Autodesk Fusion 360 part; units mm, degrees
(part 10 of 11)
  line L2802 (-0.2526, -65.3771) -> (-0.2373, -65.4277)
  line L2803 (0.0454, -65.5378) -> (0.0706, -65.5685)
  line L2804 (18.12, -173.2625) -> (18.12, -175.4997)
  line L2805 (-0.08, -80.4997) -> (-0.08, -81.4997)
  line L2806 (20.12, -54.8985) -> (20.1186, -54.7804)
  line L2807 (-0.0174, -65.4367) -> (0.0013, -65.4717)
  line L2808 (-0.0459, -65.7366) -> (1.2372, -67.0197)
  line L2809 (7.0807, -66.0997) -> (3.6807, -62.6997)
  line L2810 (19.8859, -25.7366) -> (19.9198, -25.7004)
  line L2811 (9.7152, -6.0997) -> (7.0807, -6.0997)
  line L2812 (19.7422, -174.4019) -> (18.4614, -173.1211)
  line L2813 (9.7152, -6.0997) -> (7.0807, -6.0997)
  line L2814 (19.9841, -25.6166) -> (20.012, -25.5718)
  line L2815 (18.12, -173.2625) -> (18.12, -175.4997)
  line L2816 (19.8878, -25.3633) -> (19.8993, -25.3253)
  line L2817 (19.8574, -54.5626) -> (19.8387, -54.5276)
  line L2818 (19.8993, -25.3253) -> (19.9083, -25.2866)
  line L2819 (19.9148, -25.2474) -> (19.9187, -25.2079)
  line L2820 (7.0807, -66.0997) -> (3.6807, -62.6997)
  line L2821 (20.0926, -54.6222) -> (20.0773, -54.5717)
  line L2822 (20.0773, -25.4277) -> (20.0926, -25.3771)
  line L2823 (17.92, -173.2625) -> (17.92, -175.2997)
  line L2824 (19.8738, -54.5988) -> (19.8574, -54.5626)
  line L2825 (19.7422, -174.4019) -> (18.4614, -173.1211)
  line L2826 (3.6807, -62.6997) -> (1.72, -62.6997)
  line L2827 (19.7694, -174.4308) -> (19.7422, -174.4019)
  line L2828 (19.7946, -25.5378) -> (19.8177, -25.5055)
  line L2829 (19.8878, -54.636) -> (19.8738, -54.5988)
  line L2830 (6.02, -190.1995) -> (6.02, -192.839)
  line L2831 (0.0706, -65.5685) -> (0.0978, -65.5975)
  line L2832 (12.7593, -66.0997) -> (10.127, -66.0997)
  line L2833 (20.1132, -25.2736) -> (20.1186, -25.2189)
  line L2834 (19.8387, -54.5276) -> (19.8177, -54.4938)
  line L2835 (20.0587, -25.4771) -> (20.0773, -25.4277)
  line L2836 (9.7981, -5.8997) -> (7.1635, -5.8997)
  line L2837 (16.1593, -22.6997) -> (12.7593, -26.0997)
  line L2838 (19.8878, -54.636) -> (19.8738, -54.5988)
  line L2839 (19.7946, -25.5378) -> (19.8177, -25.5055)
  line L2840 (6.02, -190.1995) -> (6.02, -192.839)
  line L2841 (1.92, -64.6997) -> (3.2765, -64.6997)
  line L2842 (19.8993, -54.674) -> (19.8878, -54.636)
  line L2843 (19.7422, -25.5975) -> (19.7694, -25.5685)
  line L2844 (0.0706, -65.5685) -> (0.0978, -65.5975)
  line L2845 (19.9187, -25.2079) -> (19.92, -25.0997)
  line L2846 (19.8177, -54.4938) -> (19.7946, -54.4616)
  arc A174 (18.4614, -173.1211) -> (18.12, -173.2625) centre (18.32, -173.2625) ccw
  line L2847 (1.72, -64.4997) -> (3.3593, -64.4997)
  line L2848 (19.8387, -54.5276) -> (19.8177, -54.4938)
  line L2849 (-0.08, -34.8997) -> (-0.08, -45.0997)
  line L2850 (19.9083, -25.2866) -> (19.9148, -25.2474)
  line L2851 (20.1186, -25.2189) -> (20.12, -25.1009)
  line L2852 (20.012, -54.4275) -> (19.9841, -54.3827)
  line L2853 (1.72, -64.4997) -> (3.3593, -64.4997)
  line L2854 (19.8859, -174.2627) -> (18.6028, -172.9797)
  line L2855 (-0.0593, -65.3253) -> (-0.0478, -65.3633)
  line L2856 (19.7694, -25.5685) -> (19.7946, -25.5378)
  line L2857 (19.7694, -174.4308) -> (19.7422, -174.4019)
  line L2858 (19.9148, -54.7519) -> (19.9083, -54.7127)
  arc A175 (18.6028, -172.9797) -> (17.92, -173.2625) centre (18.32, -173.2625) ccw
  line L2859 (3.7635, -62.4997) -> (1.92, -62.4997)
  line L2860 (3.6807, -62.6997) -> (1.72, -62.6997)
  line L2861 (20.1186, -54.7804) -> (20.1132, -54.7258)
  line L2862 (19.92, -54.8997) -> (19.9187, -54.7914)
  line L2863 (7.1635, -65.8997) -> (3.7635, -62.4997)
  line L2864 (19.8738, -54.5988) -> (19.8574, -54.5626)
  line L2865 (19.8738, -25.4005) -> (19.8878, -25.3633)
  line L2866 (20.0369, -54.4741) -> (20.012, -54.4275)
  line L2867 (20.1132, -54.7258) -> (20.1046, -54.6736)
  line L2868 (12.6765, -65.8997) -> (10.0441, -65.8997)
  line L2869 (19.8387, -25.4717) -> (19.8574, -25.4367)
  line L2870 (20.0773, -54.5717) -> (20.0587, -54.5222)
  line L2871 (13.1828, -1.9997) -> (15.22, -1.9997)
  line L2872 (19.8738, -5.4005) -> (19.8878, -5.3633)
  line L2873 (19.8878, -5.3633) -> (19.8993, -5.3253)
  line L2874 (7.0807, -46.0997) -> (3.6807, -42.6997)
  line L2875 (6.02, -7.1603) -> (6.02, -9.7998)
  line L2876 (19.9083, -25.2866) -> (19.9148, -25.2474)
  line L2877 (20.1132, -5.2736) -> (20.1184, -5.221)
  line L2878 (19.8574, -54.5626) -> (19.8387, -54.5276)
  line L2879 (5.82, -9.8826) -> (5.937, -9.9997)
  line L2880 (10.127, -166.0997) -> (9.92, -166.3066)
  line L2881 (13.82, -167.1603) -> (16.4807, -164.4997)
  line L2882 (12.6765, -14.0997) -> (16.0765, -17.4997)
  line L2883 (19.8177, -25.5055) -> (19.8387, -25.4717)
  line L2884 (6.02, -70.1995) -> (6.02, -72.839)
  line L2885 (10.0441, -165.8997) -> (9.92, -166.0238)
  arc A176 (1.3786, -6.8782) -> (1.72, -6.7368) centre (1.52, -6.7368) ccw
  line L2886 (20.0369, -5.5252) -> (20.0587, -5.4771)
  line L2887 (20.0369, -25.5252) -> (20.0587, -25.4771)
  line L2888 (14.02, -167.2432) -> (16.5635, -164.6997)
  line L2889 (6.02, -9.7998) -> (6.2199, -9.9997)
  line L2890 (19.9148, -54.7519) -> (19.9083, -54.7127)
  line L2891 (19.8993, -25.3253) -> (19.9083, -25.2866)
  line L2892 (19.8878, -5.3633) -> (19.8993, -5.3253)
  line L2893 (19.8993, -54.674) -> (19.8878, -54.636)
  line L2894 (13.82, -72.839) -> (13.82, -70.1995)
  line L2895 (6.2199, -9.9997) -> (6.02, -10.1995)
  line L2896 (5.82, -70.1167) -> (5.82, -72.7562)
  line L2897 (19.9148, -25.2474) -> (19.9187, -25.2079)
  line L2898 (9.92, -166.0238) -> (9.7959, -165.8997)
  line L2899 (13.82, -72.839) -> (13.82, -70.1995)
  line L2900 (9.92, -166.3066) -> (9.713, -166.0997)
  line L2901 (6.2199, -9.9997) -> (6.02, -10.1995)
  line L2902 (9.92, -166.3066) -> (9.713, -166.0997)
  line L2903 (20.012, -25.5718) -> (20.0369, -25.5252)
  line L2904 (19.7946, -54.4616) -> (19.7694, -54.4308)
  line L2905 (6.02, -70.1995) -> (6.02, -72.839)
  line L2906 (20.012, -5.5718) -> (20.0369, -5.5252)
  line L2907 (16.0765, -162.4997) -> (12.6765, -165.8997)
  line L2908 (19.8177, -54.4938) -> (19.7946, -54.4616)
  line L2909 (19.8993, -5.3253) -> (19.9083, -5.2866)
  line L2910 (12.7593, -166.0997) -> (10.127, -166.0997)
  line L2911 (19.8177, -25.5055) -> (19.8387, -25.4717)
  line L2912 (5.82, -7.2432) -> (5.82, -9.8826)
  line L2913 (19.8574, -25.4367) -> (19.8738, -25.4005)
  line L2914 (20.1046, -54.6736) -> (20.0926, -54.6222)
  line L2915 (19.8177, -5.5055) -> (19.8387, -5.4717)
  arc A177 (1.3786, -6.8782) -> (1.72, -6.7368) centre (1.52, -6.7368) ccw
  line L2916 (14.02, -72.7562) -> (14.02, -70.1167)
  line L2917 (20.0587, -54.5222) -> (20.0369, -54.4741)
  line L2918 (19.9533, -54.3397) -> (19.9198, -54.2989)
  line L2919 (12.7593, -166.0997) -> (10.127, -166.0997)
  line L2920 (12.7593, -66.0997) -> (10.127, -66.0997)
  line L2921 (19.9148, -5.2474) -> (19.9187, -5.2079)
  line L2922 (19.9187, -54.7914) -> (19.9148, -54.7519)
  line L2923 (16.1593, -162.6997) -> (12.7593, -166.0997)
  line L2924 (5.937, -9.9997) -> (5.82, -10.1167)
  line L2925 (14.3222, -0.1775) -> (13.0414, -1.4582)
  line L2926 (19.8574, -25.4367) -> (19.8738, -25.4005)
  line L2927 (19.9533, -25.6596) -> (19.9841, -25.6166)
  line L2928 (19.9083, -54.7127) -> (19.8993, -54.674)
  arc A178 (1.2372, -7.0197) -> (1.92, -6.7368) centre (1.52, -6.7368) ccw
  line L2929 (19.9198, -25.7004) -> (19.9533, -25.6596)
  line L2930 (19.7946, -5.5378) -> (19.8177, -5.5055)
  line L2931 (19.8387, -25.4717) -> (19.8574, -25.4367)
  line L2932 (19.7422, -54.4019) -> (18.4614, -53.1211)
  line L2933 (19.7694, -5.5685) -> (19.7946, -5.5378)
  line L2934 (19.8859, -5.7366) -> (19.9198, -5.7004)
  line L2935 (20.0587, -5.4771) -> (20.0773, -5.4277)
  line L2936 (20.0926, -25.3771) -> (20.1046, -25.3257)
  line L2937 (20.12, -45.1009) -> (20.12, -34.8985)
  line L2938 (20.0773, -5.4277) -> (20.0926, -5.3771)
  line L2939 (16.1593, -162.6997) -> (12.7593, -166.0997)
  line L2940 (19.8738, -25.4005) -> (19.8878, -25.3633)
  line L2941 (13.82, -172.839) -> (13.82, -170.1995)
  line L2942 (0.0013, -5.4717) -> (0.0223, -5.5055)
  line L2943 (19.7694, -25.5685) -> (19.7946, -25.5378)
  line L2944 (14.02, -27.2432) -> (16.5635, -24.6997)
  line L2945 (15.22, -3.3562) -> (12.6765, -5.8997)
  line L2946 (4.42, -3.439) -> (4.42, -1.7997)
  arc A179 (18.6028, -52.9797) -> (17.92, -53.2625) centre (18.32, -53.2625) ccw
  line L2947 (16.0765, -22.4997) -> (12.6765, -25.8997)
  line L2948 (19.7946, -54.4616) -> (19.7694, -54.4308)
  line L2949 (10.127, -166.0997) -> (9.92, -166.3066)
  line L2950 (20.1184, -5.221) -> (20.12, -5.1715)
  line L2951 (16.1593, -22.6997) -> (12.7593, -26.0997)
  line L2952 (18.12, -53.2625) -> (18.12, -55.4997)
  line L2953 (9.713, -173.8997) -> (9.92, -173.6927)
  line L2954 (19.8387, -5.4717) -> (19.8574, -5.4367)
  line L2955 (19.7422, -25.5975) -> (19.7694, -25.5685)
  line L2956 (19.8878, -25.3633) -> (19.8993, -25.3253)
  line L2957 (13.82, -7.1603) -> (16.4807, -4.4997)
  line L2958 (13.1828, -1.7997) -> (15.42, -1.7997)
  line L2959 (-0.172, -5.5718) -> (-0.1441, -5.6166)
  line L2960 (19.9187, -54.7914) -> (19.9148, -54.7519)
  line L2961 (14.02, -7.2432) -> (16.5635, -4.6997)
  line L2962 (17.92, -53.2625) -> (17.92, -55.2997)
  line L2963 (19.7694, -54.4308) -> (19.7422, -54.4019)
  line L2964 (12.7593, -13.8997) -> (16.1593, -17.2997)
  arc A180 (18.4614, -53.1211) -> (18.12, -53.2625) centre (18.32, -53.2625) ccw
  line L2965 (-0.08, -1.4997) -> (-0.08, -5.0997)
  line L2966 (20.1046, -25.3257) -> (20.1132, -25.2736)
  line L2967 (19.9533, -5.6596) -> (19.9841, -5.6166)
  line L2968 (-0.08, -1.4997) -> (-0.08, -5.0997)
  line L2969 (19.7694, -5.5685) -> (19.7946, -5.5378)
  line L2970 (19.7422, -54.4019) -> (18.4614, -53.1211)
  line L2971 (19.92, -54.8997) -> (19.9187, -54.7914)
  line L2972 (19.9841, -5.6166) -> (20.012, -5.5718)
  line L2973 (12.6765, -165.8997) -> (10.0441, -165.8997)
  line L2974 (13.82, -167.1603) -> (16.4807, -164.4997)
  line L2975 (6.02, -9.7998) -> (6.2199, -9.9997)
  line L2976 (19.8993, -5.3253) -> (19.9083, -5.2866)
  line L2977 (6.02, -7.1603) -> (6.02, -9.7998)
  line L2978 (20.0926, -5.3771) -> (20.1046, -5.3257)
  line L2979 (19.9187, -25.2079) -> (19.92, -25.0997)
  line L2980 (14.02, -192.7562) -> (14.02, -190.1167)
  line L2981 (19.9187, -5.2079) -> (19.92, -5.1682)
  line L2982 (20.1046, -5.3257) -> (20.1132, -5.2736)
  arc A181 (18.4614, -53.1211) -> (18.12, -53.2625) centre (18.32, -53.2625) ccw
  line L2983 (19.9148, -5.2474) -> (19.9187, -5.2079)
  line L2984 (19.8738, -5.4005) -> (19.8878, -5.3633)
  line L2985 (18.12, -53.2625) -> (18.12, -55.4997)
  line L2986 (12.7593, -13.8997) -> (16.1593, -17.2997)
  line L2987 (14.02, -170.1167) -> (13.903, -169.9997)
  line L2988 (19.9083, -5.2866) -> (19.9148, -5.2474)
  line L2989 (16.4807, -175.4997) -> (13.82, -172.839)
  line L2990 (15.42, -3.439) -> (12.7593, -6.0997)
  line L2991 (17.92, -24.6997) -> (17.92, -26.7368)
  line L2992 (-0.2373, -5.4277) -> (-0.2187, -5.4771)
  line L2993 (-0.2187, -5.4771) -> (-0.1969, -5.5252)
  line L2994 (18.4614, -26.8782) -> (19.7422, -25.5975)
  line L2995 (10.127, -173.8997) -> (12.7593, -173.8997)
  line L2996 (16.4807, -24.4997) -> (18.12, -24.4997)
  line L2997 (5.82, -190.1167) -> (5.82, -192.7562)
  line L2998 (9.92, -173.6927) -> (10.127, -173.8997)
  line L2999 (19.9083, -5.2866) -> (19.9148, -5.2474)
  line L3000 (13.6201, -169.9997) -> (13.82, -169.7998)
  arc A182 (18.12, -26.7368) -> (18.4614, -26.8782) centre (18.32, -26.7368) ccw
  line L3001 (16.5635, -24.6997) -> (17.92, -24.6997)
  line L3002 (16.4807, -175.4997) -> (13.82, -172.839)
  line L3003 (9.713, -173.8997) -> (9.92, -173.6927)
  line L3004 (13.82, -172.839) -> (13.82, -170.1995)
  line L3005 (16.4807, -4.4997) -> (18.12, -4.4997)
  arc A183 (18.12, -6.7368) -> (18.4614, -6.8782) centre (18.32, -6.7368) ccw
  line L3006 (14.3222, -0.1775) -> (13.0414, -1.4582)
  arc A184 (17.92, -26.7368) -> (18.6028, -27.0197) centre (18.32, -26.7368) ccw
  line L3007 (19.9198, -5.7004) -> (19.9533, -5.6596)
  line L3008 (4.62, -3.3562) -> (4.62, -1.9997)
  line L3009 (9.92, -173.6927) -> (10.127, -173.8997)
  line L3010 (13.82, -27.1603) -> (16.4807, -24.4997)
  arc A185 (18.12, -26.7368) -> (18.4614, -26.8782) centre (18.32, -26.7368) ccw
  line L3011 (16.4807, -24.4997) -> (18.12, -24.4997)
  line L3012 (19.8177, -5.5055) -> (19.8387, -5.4717)
  line L3013 (-0.0478, -5.3633) -> (-0.0338, -5.4005)
  line L3014 (9.92, -173.9755) -> (10.0441, -174.0997)
  line L3015 (19.8859, -54.2627) -> (18.6028, -52.9797)
  line L3016 (-0.2786, -5.2189) -> (-0.2732, -5.2736)
  line L3017 (0.0454, -5.5378) -> (0.0706, -5.5685)
  line L3018 (18.6028, -27.0197) -> (19.8859, -25.7366)
  line L3019 (-0.2526, -5.3771) -> (-0.2373, -5.4277)
  line L3020 (14.02, -172.7562) -> (14.02, -170.1167)
  line L3021 (13.6201, -169.9997) -> (13.82, -169.7998)
  line L3022 (18.4614, -26.8782) -> (19.7422, -25.5975)
  line L3023 (16.5635, -4.6997) -> (17.92, -4.6997)
  line L3024 (0.0223, -5.5055) -> (0.0454, -5.5378)
  line L3025 (20.0587, -45.4771) -> (20.0773, -45.4277)
  line L3026 (13.82, -170.1995) -> (13.6201, -169.9997)
  line L3027 (19.7694, -54.4308) -> (19.7422, -54.4019)
  line L3028 (10.0441, -174.0997) -> (12.6765, -174.0997)
  line L3029 (19.8574, -5.4367) -> (19.8738, -5.4005)
  arc A186 (17.92, -6.7368) -> (18.6028, -7.0197) centre (18.32, -6.7368) ccw
  line L3030 (19.8574, -5.4367) -> (19.8738, -5.4005)
  line L3031 (-0.0338, -5.4005) -> (-0.0174, -5.4367)
  line L3032 (0.0223, -5.5055) -> (0.0454, -5.5378)
  line L3033 (-0.2646, -5.3257) -> (-0.2526, -5.3771)
  line L3034 (-0.0338, -5.4005) -> (-0.0174, -5.4367)
  line L3035 (18.12, -24.4997) -> (18.12, -26.7368)
  line L3036 (-0.0174, -5.4367) -> (0.0013, -5.4717)
  line L3037 (13.82, -27.1603) -> (16.4807, -24.4997)
  line L3038 (19.9187, -5.2079) -> (19.92, -5.1682)
  line L3039 (1.92, -4.6997) -> (3.2765, -4.6997)
  line L3040 (-0.0593, -5.3253) -> (-0.0478, -5.3633)
  line L3041 (19.7946, -5.5378) -> (19.8177, -5.5055)
  line L3042 (18.12, -24.4997) -> (18.12, -26.7368)
  line L3043 (9.7959, -174.0997) -> (9.92, -173.9755)
  line L3044 (19.8387, -5.4717) -> (19.8574, -5.4367)
  line L3045 (16.5635, -175.2997) -> (14.02, -172.7562)
  line L3046 (13.903, -169.9997) -> (14.02, -169.8826)
  line L3047 (-0.1441, -5.6166) -> (-0.1133, -5.6596)
  line L3048 (-0.1969, -5.5252) -> (-0.172, -5.5718)
  line L3049 (13.82, -170.1995) -> (13.6201, -169.9997)
  line L3050 (-0.0593, -5.3253) -> (-0.0478, -5.3633)
  line L3051 (18.12, -4.4997) -> (18.12, -6.7368)
  line L3052 (18.12, -17.2997) -> (18.12, -22.6997)
  line L3053 (19.7422, -5.5975) -> (19.7694, -5.5685)
  line L3054 (0.0013, -5.4717) -> (0.0223, -5.5055)
  line L3055 (18.12, -162.6997) -> (16.1593, -162.6997)
  line L3056 (-0.08, -5.0997) -> (-0.0787, -5.2079)
  line L3057 (19.9198, -45.7004) -> (19.9533, -45.6596)
  line L3058 (18.4614, -6.8782) -> (19.7422, -5.5975)
  line L3059 (9.92, -13.6927) -> (10.127, -13.8997)
  line L3060 (17.92, -175.2997) -> (16.5635, -175.2997)
  line L3061 (18.12, -175.4997) -> (16.4807, -175.4997)
  line L3062 (10.127, -26.0997) -> (9.92, -26.3066)
  circle A187 centre (9.92, -169.9997) radius 2.1
  line L3063 (19.9187, -45.2079) -> (19.92, -45.0997)
  line L3064 (9.713, -13.8997) -> (9.92, -13.6927)
  line L3065 (13.82, -169.7998) -> (13.82, -167.1603)
  line L3066 (18.12, -17.2997) -> (18.12, -22.6997)
  line L3067 (19.9148, -45.2474) -> (19.9187, -45.2079)
  line L3068 (19.8177, -45.5055) -> (19.8387, -45.4717)
  line L3069 (10.127, -173.8997) -> (12.7593, -173.8997)
  line L3070 (16.0765, -17.4997) -> (17.92, -17.4997)
  line L3071 (20.1186, -45.2189) -> (20.12, -45.1009)
  line L3072 (18.12, -175.4997) -> (16.4807, -175.4997)
  line L3073 (16.4807, -164.4997) -> (18.12, -164.4997)
  line L3074 (0.0706, -5.5685) -> (0.0978, -5.5975)
  circle A188 centre (9.92, -169.9997) radius 2.1
  line L3075 (-0.0683, -5.2866) -> (-0.0593, -5.3253)
  line L3076 (9.713, -13.8997) -> (9.92, -13.6927)
  line L3077 (-0.0787, -5.2079) -> (-0.0748, -5.2474)
  line L3078 (7.0807, -13.8997) -> (9.713, -13.8997)
  line L3079 (-0.08, -5.0997) -> (-0.0787, -5.2079)
  arc A189 (18.12, -6.7368) -> (18.4614, -6.8782) centre (18.32, -6.7368) ccw
  line L3080 (12.6765, -25.8997) -> (10.0441, -25.8997)
  line L3081 (19.8387, -45.4717) -> (19.8574, -45.4367)
  line L3082 (16.5635, -164.6997) -> (17.92, -164.6997)
  line L3083 (18.12, -22.6997) -> (16.1593, -22.6997)
  line L3084 (13.82, -169.7998) -> (13.82, -167.1603)
  line L3085 (-0.1133, -5.6596) -> (-0.0798, -5.7004)
  line L3086 (16.1593, -17.2997) -> (18.12, -17.2997)
  line L3087 (0.0454, -5.5378) -> (0.0706, -5.5685)
  line L3088 (17.92, -4.6997) -> (17.92, -6.7368)
  line L3089 (9.92, -13.9755) -> (10.0441, -14.0997)
  line L3090 (18.4614, -6.8782) -> (19.7422, -5.5975)
  line L3091 (16.4807, -4.4997) -> (18.12, -4.4997)
  line L3092 (19.7422, -5.5975) -> (19.7694, -5.5685)
  line L3093 (18.12, -4.4997) -> (18.12, -6.7368)
  line L3094 (-0.0174, -5.4367) -> (0.0013, -5.4717)
  line L3095 (19.7694, -45.5685) -> (19.7946, -45.5378)
  line L3096 (18.12, -22.6997) -> (16.1593, -22.6997)
  line L3097 (17.92, -17.4997) -> (17.92, -22.4997)
  line L3098 (16.1593, -17.2997) -> (18.12, -17.2997)
  line L3099 (10.127, -26.0997) -> (9.92, -26.3066)
  line L3100 (19.9187, -45.2079) -> (19.92, -45.0997)
  line L3101 (7.1635, -14.0997) -> (9.7959, -14.0997)
  line L3102 (19.8878, -45.3633) -> (19.8993, -45.3253)
  line L3103 (14.02, -169.8826) -> (14.02, -167.2432)
  line L3104 (-0.0748, -5.2474) -> (-0.0683, -5.2866)
  line L3105 (17.92, -22.4997) -> (16.0765, -22.4997)
  line L3106 (-0.0478, -5.3633) -> (-0.0338, -5.4005)
  line L3107 (12.7593, -26.0997) -> (10.127, -26.0997)
  line L3108 (20.012, -45.5718) -> (20.0369, -45.5252)
  line L3109 (9.7959, -25.8997) -> (7.1635, -25.8997)
  line L3110 (18.6028, -7.0197) -> (19.8859, -5.7366)
  line L3111 (19.9083, -45.2866) -> (19.9148, -45.2474)
  line L3112 (0.0706, -5.5685) -> (0.0978, -5.5975)
  line L3113 (19.8387, -45.4717) -> (19.8574, -45.4367)
  line L3114 (18.12, -162.6997) -> (16.1593, -162.6997)
  line L3115 (10.0441, -14.0997) -> (12.6765, -14.0997)
  line L3116 (16.4807, -164.4997) -> (18.12, -164.4997)
  line L3117 (9.92, -26.3066) -> (9.713, -26.0997)
  line L3118 (9.92, -26.0238) -> (9.7959, -25.8997)
  line L3119 (19.9533, -45.6596) -> (19.9841, -45.6166)
  line L3120 (-0.2732, -5.2736) -> (-0.2646, -5.3257)
  line L3121 (17.92, -162.4997) -> (16.0765, -162.4997)
  line L3122 (20.0369, -45.5252) -> (20.0587, -45.4771)
  line L3123 (-0.0798, -5.7004) -> (-0.0459, -5.7366)
  line L3124 (10.0441, -25.8997) -> (9.92, -26.0238)
  line L3125 (7.0807, -93.8997) -> (9.713, -93.8997)
  line L3126 (14.483, -140.0623) -> (14.4479, -140.081)
  line L3127 (14.2601, -139.9663) -> (14.2193, -139.9999)
  line L3128 (14.5191, -140.0459) -> (14.483, -140.0623)
  line L3129 (14.492, -140.1569) -> (14.5425, -140.1723)
  line L3130 (14.2601, -140.033) -> (14.303, -140.0637)
  line L3131 (9.92, -93.6927) -> (10.127, -93.8997)
  line L3132 (14.3512, -140.1503) -> (14.3222, -140.1775)
  line L3133 (14.5191, -140.0459) -> (14.483, -140.0623)
  line L3134 (9.92, -93.6927) -> (10.127, -93.8997)
  line L3135 (14.4142, -140.102) -> (14.3819, -140.1251)
  line L3136 (14.3819, -140.1251) -> (14.3512, -140.1503)
  line L3137 (10.0441, -105.8997) -> (9.92, -106.0238)
  line L3138 (10.127, -93.8997) -> (12.7593, -93.8997)
  line L3139 (16.1593, -102.6997) -> (12.7593, -106.0997)
  line L3140 (16.4807, -95.4997) -> (13.82, -92.839)
  line L3141 (14.3945, -140.1165) -> (14.4426, -140.1383)
  line L3142 (14.4142, -140.102) -> (14.3819, -140.1251)
  line L3143 (14.4479, -140.081) -> (14.4142, -140.102)
  line L3144 (14.3479, -140.0916) -> (14.3945, -140.1165)
  line L3145 (14.2193, -139.9995) -> (14.2601, -140.033)
  line L3146 (14.5563, -140.0319) -> (14.5191, -140.0459)
  line L3147 (14.5563, -140.0319) -> (14.5191, -140.0459)
  line L3148 (16.1593, -102.6997) -> (12.7593, -106.0997)
  line L3149 (14.6987, -140.198) -> (14.7482, -140.1997)
  line L3150 (14.4479, -140.081) -> (14.4142, -140.102)
  line L3151 (14.4426, -140.1383) -> (14.492, -140.1569)
  line L3152 (14.303, -140.0637) -> (14.3479, -140.0916)
  line L3153 (14.3819, -140.1251) -> (14.3512, -140.1503)
  line L3154 (14.483, -140.0623) -> (14.4479, -140.081)
  line L3155 (14.5425, -140.1723) -> (14.594, -140.1843)
  line L3156 (14.3512, -140.1503) -> (14.3222, -140.1775)
  line L3157 (14.303, -79.9356) -> (14.2601, -79.9663)
  line L3158 (14.492, -79.8424) -> (14.4426, -79.861)
  line L3159 (14.4479, -80.081) -> (14.4142, -80.102)
  line L3160 (13.82, -129.7998) -> (13.82, -127.1603)
  line L3161 (14.303, -80.0637) -> (14.3479, -80.0916)
  line L3162 (16.4807, -124.4997) -> (18.12, -124.4997)
  line L3163 (14.4142, -80.102) -> (14.3819, -80.1251)
  line L3164 (13.903, -129.9997) -> (14.02, -129.8826)
  line L3165 (16.4807, -124.4997) -> (18.12, -124.4997)
  line L3166 (14.483, -79.9371) -> (14.5191, -79.9534)
  line L3167 (20.12, -165.1009) -> (20.12, -154.8985)
  line L3168 (13.6201, -129.9997) -> (13.82, -129.7998)
  line L3169 (10.127, -126.0997) -> (9.92, -126.3066)
  line L3170 (13.82, -129.7998) -> (13.82, -127.1603)
  line L3171 (14.3512, -79.849) -> (14.3819, -79.8742)
  line L3172 (14.4479, -79.9183) -> (14.483, -79.9371)
  line L3173 (13.6201, -129.9997) -> (13.82, -129.7998)
  line L3174 (14.02, -130.1167) -> (13.903, -129.9997)
  line L3175 (14.3512, -80.1503) -> (14.3222, -80.1775)
  line L3176 (14.5191, -80.0459) -> (14.483, -80.0623)
  line L3177 (14.3819, -80.1251) -> (14.3512, -80.1503)
  line L3178 (12.7593, -126.0997) -> (10.127, -126.0997)
  line L3179 (14.3819, -80.1251) -> (14.3512, -80.1503)
  line L3180 (9.92, -126.3066) -> (9.713, -126.0997)
  line L3181 (14.4142, -79.8974) -> (14.4479, -79.9183)
  line L3182 (9.92, -126.0238) -> (9.7959, -125.8997)
  line L3183 (14.7482, -80.1997) -> (18.42, -80.1997)
  line L3184 (12.7593, -133.8997) -> (15.42, -136.5603)
  arc A190 (19.42, -79.9997) -> (19.92, -79.4997) centre (19.42, -79.4997) ccw
  line L3185 (19.8859, -134.2627) -> (18.6028, -132.9797)
  line L3186 (9.7152, -133.8997) -> (9.92, -133.6949)
  line L3187 (10.127, -133.8997) -> (12.7593, -133.8997)
  arc A191 (20.12, -80.4997) -> (19.42, -79.7997) centre (19.42, -80.4997) ccw
  line L3188 (10.0448, -134.0997) -> (12.6765, -134.0997)
  line L3189 (19.7694, -134.4308) -> (19.7422, -134.4019)
  line L3190 (13.82, -132.839) -> (13.82, -130.1995)
  line L3191 (9.92, -133.6949) -> (10.127, -133.8997)
  line L3192 (12.7593, -133.8997) -> (15.42, -136.5603)
  line L3193 (9.92, -133.6949) -> (10.127, -133.8997)
  arc A192 (19.92, -80.4997) -> (19.42, -79.9997) centre (19.42, -80.4997) ccw
  line L3194 (13.82, -132.839) -> (13.82, -130.1995)
  line L3195 (12.6765, -134.0997) -> (15.22, -136.6432)
  line L3196 (18.42, -80.1997) -> (19.42, -80.1997)
  line L3197 (9.7981, -134.0997) -> (9.9208, -133.977)
  line L3198 (18.42, -79.9997) -> (14.7514, -79.9997)
  line L3199 (16.4807, -135.4997) -> (13.82, -132.839)
  line L3200 (19.42, -79.7997) -> (18.42, -79.7997)
  line L3201 (19.42, -79.9997) -> (18.42, -79.9997)
  arc A193 (19.42, -80.1997) -> (20.12, -79.4997) centre (19.42, -79.4997) ccw
  line L3202 (10.127, -133.8997) -> (12.7593, -133.8997)
  line L3203 (16.4807, -135.4997) -> (13.82, -132.839)
  line L3204 (9.9208, -133.977) -> (10.0448, -134.0997)
  line L3205 (18.42, -79.7997) -> (14.7482, -79.7997)
  arc A194 (19.42, -79.9997) -> (19.92, -79.4997) centre (19.42, -79.4997) ccw
  line L3206 (14.7514, -79.9997) -> (18.42, -79.9997)
  arc A195 (19.92, -80.4997) -> (19.42, -79.9997) centre (19.42, -80.4997) ccw
  line L3207 (18.42, -79.9997) -> (19.42, -79.9997)
  line L3208 (19.42, -79.9997) -> (18.42, -79.9997)
  line L3209 (18.42, -79.9997) -> (19.42, -79.9997)
  line L3210 (16.5635, -135.2997) -> (14.02, -132.7562)
  line L3211 (14.7514, -79.9997) -> (18.42, -79.9997)
  line L3212 (9.7152, -133.8997) -> (9.92, -133.6949)
  line L3213 (18.42, -79.9997) -> (14.7514, -79.9997)
  line L3214 (20.1132, -125.2736) -> (20.1186, -125.2189)
  line L3215 (19.8993, -125.3253) -> (19.9083, -125.2866)
  line L3216 (20.0926, -125.3771) -> (20.1046, -125.3257)
  line L3217 (20.1186, -125.2189) -> (20.12, -125.1009)
  line L3218 (20.012, -125.5718) -> (20.0369, -125.5252)
  line L3219 (19.7694, -125.5685) -> (19.7946, -125.5378)
  line L3220 (19.7694, -125.5685) -> (19.7946, -125.5378)
  line L3221 (19.7946, -125.5378) -> (19.8177, -125.5055)
  line L3222 (19.8993, -125.3253) -> (19.9083, -125.2866)
  line L3223 (19.8878, -125.3633) -> (19.8993, -125.3253)
  line L3224 (19.9187, -125.2079) -> (19.92, -125.0997)
  line L3225 (20.0587, -125.4771) -> (20.0773, -125.4277)
  line L3226 (19.9533, -125.6596) -> (19.9841, -125.6166)
  line L3227 (20.1046, -125.3257) -> (20.1132, -125.2736)
  line L3228 (14.6987, -79.8013) -> (14.6461, -79.8065)
  line L3229 (18.12, -157.2997) -> (18.12, -162.6997)
  line L3230 (19.9083, -125.2866) -> (19.9148, -125.2474)
  line L3231 (14.6722, -80.0049) -> (14.633, -80.0113)
  line L3232 (20.0369, -125.5252) -> (20.0587, -125.4771)
  line L3233 (19.8859, -125.7366) -> (19.9198, -125.7004)
  line L3234 (14.594, -79.8151) -> (14.5425, -79.8271)
  line L3235 (14.633, -79.988) -> (14.6722, -79.9945)
  line L3236 (19.9148, -125.2474) -> (19.9187, -125.2079)
  line L3237 (19.9187, -125.2079) -> (19.92, -125.0997)
  line L3238 (14.5563, -79.9674) -> (14.5943, -79.979)
  line L3239 (14.7117, -80.001) -> (14.6722, -80.0049)
  line L3240 (19.8738, -125.4005) -> (19.8878, -125.3633)
  line L3241 (19.8574, -125.4367) -> (19.8738, -125.4005)
  line L3242 (19.9083, -125.2866) -> (19.9148, -125.2474)
  line L3243 (14.5425, -80.1723) -> (14.594, -80.1843)
  line L3244 (19.9841, -125.6166) -> (20.012, -125.5718)
  line L3245 (19.8574, -125.4367) -> (19.8738, -125.4005)
  line L3246 (14.6461, -80.1929) -> (14.6987, -80.198)
  line L3247 (19.8387, -125.4717) -> (19.8574, -125.4367)
  line L3248 (19.8878, -125.3633) -> (19.8993, -125.3253)
  line L3249 (19.8177, -125.5055) -> (19.8387, -125.4717)
  line L3250 (19.7946, -125.5378) -> (19.8177, -125.5055)
  line L3251 (19.8738, -125.4005) -> (19.8878, -125.3633)
  line L3252 (19.8177, -125.5055) -> (19.8387, -125.4717)
  line L3253 (20.0773, -125.4277) -> (20.0926, -125.3771)
  line L3254 (19.8387, -125.4717) -> (19.8574, -125.4367)
  line L3255 (19.9198, -125.7004) -> (19.9533, -125.6596)
  line L3256 (19.9148, -125.2474) -> (19.9187, -125.2079)
  line L3257 (14.6722, -80.0049) -> (14.633, -80.0113)
  line L3258 (18.4614, -126.8782) -> (19.7422, -125.5975)
  line L3259 (14.5943, -79.979) -> (14.633, -79.988)
  line L3260 (14.6461, -79.8065) -> (14.594, -79.8151)
  line L3261 (14.594, -80.1843) -> (14.6461, -80.1929)
  line L3262 (18.4614, -126.8782) -> (19.7422, -125.5975)
  line L3263 (14.633, -79.988) -> (14.6722, -79.9945)
  arc A196 (18.12, -126.7368) -> (18.4614, -126.8782) centre (18.32, -126.7368) ccw
  line L3264 (14.5943, -79.979) -> (14.633, -79.988)
  line L3265 (14.6722, -79.9945) -> (14.7117, -79.9984)
  arc A197 (17.92, -126.7368) -> (18.6028, -127.0197) centre (18.32, -126.7368) ccw
  line L3266 (14.5563, -79.9674) -> (14.5943, -79.979)
  line L3267 (14.6722, -79.9945) -> (14.7117, -79.9984)
  line L3268 (14.633, -80.0113) -> (14.5943, -80.0203)
  arc A198 (18.12, -126.7368) -> (18.4614, -126.8782) centre (18.32, -126.7368) ccw
  line L3269 (14.5943, -80.0203) -> (14.5563, -80.0319)
  line L3270 (18.12, -124.4997) -> (18.12, -126.7368)
  line L3271 (14.7117, -80.001) -> (14.6722, -80.0049)
  line L3272 (18.12, -124.4997) -> (18.12, -126.7368)
  line L3273 (17.92, -124.6997) -> (17.92, -126.7368)
  line L3274 (14.5943, -80.0203) -> (14.5563, -80.0319)
  line L3275 (10.127, -126.0997) -> (9.92, -126.3066)
  line L3276 (14.2193, -79.9995) -> (14.2601, -80.033)
  line L3277 (10.0441, -125.8997) -> (9.92, -126.0238)
  line L3278 (14.2601, -79.9663) -> (14.2193, -79.9999)
  line L3279 (14.483, -79.9371) -> (14.5191, -79.9534)
  line L3280 (13.82, -127.1603) -> (16.4807, -124.4997)
  line L3281 (14.3945, -79.8828) -> (14.3479, -79.9077)
  line L3282 (19.7422, -125.5975) -> (19.7694, -125.5685)
  line L3283 (19.7422, -125.5975) -> (19.7694, -125.5685)
  line L3284 (14.633, -80.0113) -> (14.5943, -80.0203)
  line L3285 (12.6765, -125.8997) -> (10.0441, -125.8997)
  line L3286 (18.6028, -127.0197) -> (19.8859, -125.7366)
  line L3287 (13.82, -127.1603) -> (16.4807, -124.4997)
  line L3288 (14.02, -127.2432) -> (16.5635, -124.6997)
  line L3289 (14.4479, -79.9183) -> (14.483, -79.9371)
  line L3290 (14.02, -129.8826) -> (14.02, -127.2432)
  line L3291 (14.3479, -80.0916) -> (14.3945, -80.1165)
  line L3292 (9.92, -126.3066) -> (9.713, -126.0997)
  line L3293 (12.7593, -126.0997) -> (10.127, -126.0997)
  line L3294 (12.7593, -106.0997) -> (10.127, -106.0997)
  line L3295 (10.127, -106.0997) -> (9.92, -106.3066)
  line L3296 (14.6722, -140.0049) -> (14.633, -140.0113)
  line L3297 (9.713, -106.0997) -> (7.0807, -106.0997)
  line L3298 (14.6722, -139.9945) -> (14.7117, -139.9984)
  line L3299 (14.7117, -140.001) -> (14.6722, -140.0049)
  line L3300 (14.594, -140.1843) -> (14.6461, -140.1929)
  line L3301 (9.713, -93.8997) -> (9.92, -93.6927)
  line L3302 (14.5943, -139.979) -> (14.633, -139.988)
  line L3303 (14.02, -107.2432) -> (16.5635, -104.6997)
  line L3304 (14.6461, -140.1929) -> (14.6987, -140.198)
  line L3305 (14.7514, -139.9997) -> (18.42, -139.9997)
  line L3306 (10.0441, -94.0997) -> (12.6765, -94.0997)
  line L3307 (9.713, -93.8997) -> (9.92, -93.6927)
  line L3308 (9.7959, -94.0997) -> (9.92, -93.9755)
  line L3309 (7.1635, -94.0997) -> (9.7959, -94.0997)
  line L3310 (12.6765, -105.8997) -> (10.0441, -105.8997)
  line L3311 (14.633, -140.0113) -> (14.5943, -140.0203)
  line L3312 (14.7117, -140.001) -> (14.6722, -140.0049)
  line L3313 (12.7593, -93.8997) -> (16.1593, -97.2997)
  line L3314 (12.7593, -106.0997) -> (10.127, -106.0997)
  line L3315 (14.5563, -139.9674) -> (14.5943, -139.979)
  line L3316 (10.127, -106.0997) -> (9.92, -106.3066)
  line L3317 (16.5635, -95.2997) -> (14.02, -92.7562)
  line L3318 (14.6722, -139.9945) -> (14.7117, -139.9984)
  line L3319 (14.633, -139.988) -> (14.6722, -139.9945)
  line L3320 (9.7959, -105.8997) -> (7.1635, -105.8997)
  line L3321 (9.92, -106.0238) -> (9.7959, -105.8997)
  line L3322 (14.6722, -140.0049) -> (14.633, -140.0113)
  line L3323 (14.5563, -139.9674) -> (14.5943, -139.979)
  line L3324 (7.0807, -93.8997) -> (9.713, -93.8997)
  line L3325 (9.92, -93.9755) -> (10.0441, -94.0997)
  line L3326 (14.633, -140.0113) -> (14.5943, -140.0203)
  line L3327 (16.4807, -95.4997) -> (13.82, -92.839)
  line L3328 (14.5943, -139.979) -> (14.633, -139.988)
  line L3329 (14.633, -139.988) -> (14.6722, -139.9945)
  line L3330 (12.6765, -94.0997) -> (16.0765, -97.4997)
  line L3331 (14.5943, -140.0203) -> (14.5563, -140.0319)
  line L3332 (10.127, -93.8997) -> (12.7593, -93.8997)
  line L3333 (12.7593, -93.8997) -> (16.1593, -97.2997)
  line L3334 (9.92, -106.3066) -> (9.713, -106.0997)
  line L3335 (14.5943, -140.0203) -> (14.5563, -140.0319)
  line L3336 (16.0765, -102.4997) -> (12.6765, -105.8997)
  line L3337 (13.82, -107.1603) -> (16.4807, -104.4997)
  line L3338 (3.3593, -155.4997) -> (1.72, -155.4997)
  line L3339 (1.72, -157.2997) -> (3.6807, -157.2997)
  line L3340 (1.92, -157.4997) -> (3.7635, -157.4997)
  line L3341 (12.7593, -153.8997) -> (16.1593, -157.2997)
  line L3342 (12.6765, -154.0997) -> (16.0765, -157.4997)
  line L3343 (18.12, -153.2625) -> (18.12, -155.4997)
  line L3344 (0.0454, -154.4616) -> (0.0223, -154.4938)
  line L3345 (1.72, -157.2997) -> (3.6807, -157.2997)
  line L3346 (3.3593, -155.4997) -> (1.72, -155.4997)
  line L3347 (3.2765, -155.2997) -> (1.92, -155.2997)
  line L3348 (16.4807, -155.4997) -> (13.82, -152.839)
  line L3349 (14.7117, -139.9984) -> (14.7514, -139.9997)
  line L3350 (17.92, -95.2997) -> (16.5635, -95.2997)
  line L3351 (13.82, -107.1603) -> (16.4807, -104.4997)
  line L3352 (19.42, -139.9997) -> (18.42, -139.9997)
  line L3353 (18.42, -139.9997) -> (19.42, -139.9997)
  line L3354 (16.5635, -104.6997) -> (17.92, -104.6997)
  line L3355 (18.42, -140.1997) -> (19.42, -140.1997)
  line L3356 (16.0765, -97.4997) -> (17.92, -97.4997)
  line L3357 (18.6028, -147.0197) -> (19.8859, -145.7366)
  line L3358 (9.92, -106.3066) -> (9.713, -106.0997)
  line L3359 (19.42, -139.9997) -> (18.42, -139.9997)
  line L3360 (16.1593, -97.2997) -> (18.12, -97.2997)
  line L3361 (9.713, -106.0997) -> (7.0807, -106.0997)
  line L3362 (18.4614, -146.8782) -> (19.7422, -145.5975)
  line L3363 (18.12, -95.4997) -> (16.4807, -95.4997)
  line L3364 (14.7514, -139.9997) -> (14.7117, -140.001)
  line L3365 (14.7117, -139.9984) -> (14.7514, -139.9997)
  line L3366 (16.1593, -97.2997) -> (18.12, -97.2997)
  line L3367 (14.7514, -139.9997) -> (14.7117, -140.001)
  line L3368 (18.42, -139.9997) -> (19.42, -139.9997)
  line L3369 (17.92, -102.4997) -> (16.0765, -102.4997)
  line L3370 (16.4807, -104.4997) -> (18.12, -104.4997)
  line L3371 (16.4807, -104.4997) -> (18.12, -104.4997)
  line L3372 (18.12, -95.4997) -> (16.4807, -95.4997)
  line L3373 (18.4614, -146.8782) -> (19.7422, -145.5975)
  line L3374 (19.42, -139.7997) -> (18.42, -139.7997)
  line L3375 (1.72, -106.7368) -> (1.72, -104.4997)
  line L3376 (14.6461, -139.8065) -> (14.594, -139.8151)
  line L3377 (1.72, -104.4997) -> (3.3593, -104.4997)
  line L3378 (20.12, -139.4997) -> (20.12, -138.4997)
  line L3379 (14.594, -139.8151) -> (14.5425, -139.8271)
  line L3380 (18.12, -102.6997) -> (16.1593, -102.6997)
  line L3381 (18.12, -102.6997) -> (16.1593, -102.6997)
  line L3382 (18.42, -139.7997) -> (14.7482, -139.7997)
  line L3383 (14.6987, -139.8013) -> (14.6461, -139.8065)
  line L3384 (19.92, -139.4997) -> (19.92, -138.4997)
  arc A199 (1.3786, -106.8782) -> (1.72, -106.7368) centre (1.52, -106.7368) ccw
  line L3385 (19.92, -139.4997) -> (19.92, -138.4997)
  arc A200 (1.3786, -106.8782) -> (1.72, -106.7368) centre (1.52, -106.7368) ccw
  line L3386 (16.4807, -64.4997) -> (18.12, -64.4997)
  line L3387 (20.12, -138.4997) -> (20.12, -134.8278)
  line L3388 (16.5635, -64.6997) -> (17.92, -64.6997)
  line L3389 (19.7422, -65.5975) -> (19.7694, -65.5685)
  line L3390 (19.8177, -65.5055) -> (19.8387, -65.4717)
  line L3391 (19.9148, -65.2474) -> (19.9187, -65.2079)
  line L3392 (19.9083, -65.2866) -> (19.9148, -65.2474)
  line L3393 (19.8574, -65.4367) -> (19.8738, -65.4005)
  line L3394 (4.62, -137.9997) -> (4.62, -136.6432)
  line L3395 (4.42, -138.1997) -> (4.42, -136.5603)
  line L3396 (20.012, -65.5718) -> (20.0369, -65.5252)
  line L3397 (19.8878, -65.3633) -> (19.8993, -65.3253)
  line L3398 (20.0369, -65.5252) -> (20.0587, -65.4771)
  line L3399 (19.8859, -65.7366) -> (19.9198, -65.7004)
  line L3400 (15.22, -136.6432) -> (15.22, -137.9997)
  line L3401 (-0.08, -134.8997) -> (-0.08, -138.4997)
  line L3402 (20.1046, -65.3257) -> (20.1132, -65.2736)
  line L3403 (19.92, -138.4997) -> (19.92, -134.8311)
  line L3404 (15.42, -136.5603) -> (15.42, -138.1997)
  line L3405 (19.8574, -65.4367) -> (19.8738, -65.4005)
  line L3406 (19.7946, -65.5378) -> (19.8177, -65.5055)
  line L3407 (14.02, -67.2432) -> (16.5635, -64.6997)
  line L3408 (19.7422, -65.5975) -> (19.7694, -65.5685)
  line L3409 (19.8387, -65.4717) -> (19.8574, -65.4367)
  line L3410 (19.9083, -165.2866) -> (19.9148, -165.2474)
  line L3411 (13.82, -67.1603) -> (16.4807, -64.4997)
  line L3412 (19.9841, -65.6166) -> (20.012, -65.5718)
  line L3413 (20.0587, -65.4771) -> (20.0773, -65.4277)
  line L3414 (19.8738, -65.4005) -> (19.8878, -65.3633)
  line L3415 (18.6028, -67.0197) -> (19.8859, -65.7366)
  line L3416 (19.7694, -65.5685) -> (19.7946, -65.5378)
  line L3417 (19.9198, -65.7004) -> (19.9533, -65.6596)
  line L3418 (19.8993, -65.3253) -> (19.9083, -65.2866)
  line L3419 (19.9187, -65.2079) -> (19.92, -65.0997)
  line L3420 (16.4807, -64.4997) -> (18.12, -64.4997)
  line L3421 (19.7694, -65.5685) -> (19.7946, -65.5378)
  line L3422 (19.9148, -65.2474) -> (19.9187, -65.2079)
  line L3423 (19.8878, -65.3633) -> (19.8993, -65.3253)
  line L3424 (18.4614, -66.8782) -> (19.7422, -65.5975)
  line L3425 (18.4614, -66.8782) -> (19.7422, -65.5975)
  line L3426 (19.9148, -165.2474) -> (19.9187, -165.2079)
  line L3427 (18.12, -62.6997) -> (16.1593, -62.6997)
  line L3428 (16.0765, -62.4997) -> (12.6765, -65.8997)
  line L3429 (19.9533, -165.6596) -> (19.9841, -165.6166)
  line L3430 (19.7946, -165.5378) -> (19.8177, -165.5055)
  line L3431 (19.8993, -165.3253) -> (19.9083, -165.2866)
  line L3432 (18.12, -64.4997) -> (18.12, -66.7368)
  line L3433 (20.1132, -165.2736) -> (20.1186, -165.2189)
  line L3434 (13.82, -67.1603) -> (16.4807, -64.4997)
  line L3435 (20.1186, -165.2189) -> (20.12, -165.1009)
  line L3436 (19.8387, -165.4717) -> (19.8574, -165.4367)
  line L3437 (18.12, -62.6997) -> (16.1593, -62.6997)
  line L3438 (18.12, -64.4997) -> (18.12, -66.7368)
  line L3439 (17.92, -62.4997) -> (16.0765, -62.4997)
  line L3440 (19.8738, -165.4005) -> (19.8878, -165.3633)
  line L3441 (19.9187, -165.2079) -> (19.92, -165.0997)
  line L3442 (19.8177, -165.5055) -> (19.8387, -165.4717)
  line L3443 (19.9148, -165.2474) -> (19.9187, -165.2079)
  line L3444 (17.92, -64.6997) -> (17.92, -66.7368)
  line L3445 (16.1593, -62.6997) -> (12.7593, -66.0997)
  line L3446 (16.1593, -62.6997) -> (12.7593, -66.0997)
  line L3447 (19.8859, -165.7366) -> (19.9198, -165.7004)
  line L3448 (19.7946, -165.5378) -> (19.8177, -165.5055)
  line L3449 (19.9841, -165.6166) -> (20.012, -165.5718)
  line L3450 (20.0369, -165.5252) -> (20.0587, -165.4771)
  line L3451 (19.7694, -165.5685) -> (19.7946, -165.5378)
  line L3452 (20.012, -165.5718) -> (20.0369, -165.5252)
  line L3453 (19.8387, -165.4717) -> (19.8574, -165.4367)
  line L3454 (20.0926, -165.3771) -> (20.1046, -165.3257)
  line L3455 (19.9198, -165.7004) -> (19.9533, -165.6596)
  line L3456 (19.8177, -165.5055) -> (19.8387, -165.4717)
  line L3457 (3.2765, -64.6997) -> (5.82, -67.2432)
  line L3458 (20.0587, -165.4771) -> (20.0773, -165.4277)
  line L3459 (9.92, -66.0238) -> (9.7959, -65.8997)
  line L3460 (20.1046, -165.3257) -> (20.1132, -165.2736)
  line L3461 (10.127, -66.0997) -> (9.92, -66.3066)
  line L3462 (9.713, -66.0997) -> (7.0807, -66.0997)
  line L3463 (20.0773, -165.4277) -> (20.0926, -165.3771)
  line L3464 (19.8878, -165.3633) -> (19.8993, -165.3253)
  line L3465 (19.8993, -165.3253) -> (19.9083, -165.2866)
  line L3466 (19.9187, -165.2079) -> (19.92, -165.0997)
  line L3467 (6.02, -69.7998) -> (6.2199, -69.9997)
  line L3468 (6.02, -67.1603) -> (6.02, -69.7998)
  arc A201 (18.12, -166.7368) -> (18.4614, -166.8782) centre (18.32, -166.7368) ccw
  line L3469 (18.12, -164.4997) -> (18.12, -166.7368)
  line L3470 (3.3593, -64.4997) -> (6.02, -67.1603)
  line L3471 (9.7959, -65.8997) -> (7.1635, -65.8997)
  line L3472 (19.8878, -165.3633) -> (19.8993, -165.3253)
  line L3473 (10.127, -66.0997) -> (9.92, -66.3066)
  line L3474 (19.8738, -165.4005) -> (19.8878, -165.3633)
  line L3475 (19.7694, -165.5685) -> (19.7946, -165.5378)
  line L3476 (19.8574, -165.4367) -> (19.8738, -165.4005)
  line L3477 (9.92, -66.3066) -> (9.713, -66.0997)
  circle A202 centre (9.92, -69.9997) radius 2.1
  line L3478 (19.8574, -165.4367) -> (19.8738, -165.4005)
  line L3479 (10.0441, -65.8997) -> (9.92, -66.0238)
  line L3480 (6.2199, -69.9997) -> (6.02, -70.1995)
  line L3481 (19.9083, -165.2866) -> (19.9148, -165.2474)
  line L3482 (6.02, -67.1603) -> (6.02, -69.7998)
  line L3483 (9.713, -66.0997) -> (7.0807, -66.0997)
  line L3484 (6.02, -69.7998) -> (6.2199, -69.9997)
  circle A203 centre (9.92, -69.9997) radius 2.1
  line L3485 (5.937, -69.9997) -> (5.82, -70.1167)
  line L3486 (18.4614, -166.8782) -> (19.7422, -165.5975)
  line L3487 (5.82, -67.2432) -> (5.82, -69.8826)
  arc A204 (1.3786, -66.8782) -> (1.72, -66.7368) centre (1.52, -66.7368) ccw
  line L3488 (18.12, -164.4997) -> (18.12, -166.7368)
  line L3489 (1.72, -66.7368) -> (1.72, -64.4997)
  arc A205 (17.92, -166.7368) -> (18.6028, -167.0197) centre (18.32, -166.7368) ccw
  line L3490 (19.7422, -165.5975) -> (19.7694, -165.5685)
  line L3491 (5.82, -69.8826) -> (5.937, -69.9997)
  line L3492 (17.92, -164.6997) -> (17.92, -166.7368)
  arc A206 (18.12, -166.7368) -> (18.4614, -166.8782) centre (18.32, -166.7368) ccw
  line L3493 (17.92, -157.4997) -> (17.92, -162.4997)
  line L3494 (18.4614, -166.8782) -> (19.7422, -165.5975)
  line L3495 (20, 0) -> (-3, 0)
  line L3496 (18.6028, -167.0197) -> (19.8859, -165.7366)
  line L3497 (-0.08, -154.8997) -> (-0.08, -165.0997)
  line L3498 (18.12, -57.2997) -> (18.12, -62.6997)
  line L3499 (-0.28, -54.8985) -> (-0.28, -65.1009)
  line L3500 (19.7422, -165.5975) -> (19.7694, -165.5685)
  line L3501 (6.2199, -69.9997) -> (6.02, -70.1995)
  line L3502 (3.3593, -64.4997) -> (6.02, -67.1603)
  line L3503 (9.92, -66.3066) -> (9.713, -66.0997)
  line L3504 (0.0978, -65.5975) -> (1.3786, -66.8782)
  line L3505 (19.92, -165.0997) -> (19.92, -154.8997)
  line L3506 (1.72, -66.7368) -> (1.72, -64.4997)
  arc A207 (1.3786, -66.8782) -> (1.72, -66.7368) centre (1.52, -66.7368) ccw
  line L3507 (19.92, -165.0997) -> (19.92, -154.8997)
  line L3508 (1.72, -62.6997) -> (1.72, -57.2997)
  line L3509 (19.8878, -174.636) -> (19.8738, -174.5988)
  line L3510 (19.9148, -174.7519) -> (19.9083, -174.7127)
  line L3511 (19.9533, -174.3397) -> (19.9198, -174.2989)
  line L3512 (-0.1441, -65.6166) -> (-0.1133, -65.6596)
  line L3513 (0.0978, -65.5975) -> (1.3786, -66.8782)
  line L3514 (19.7946, -174.4616) -> (19.7694, -174.4308)
  line L3515 (19.9187, -174.7914) -> (19.9148, -174.7519)
  line L3516 (19.9083, -174.7127) -> (19.8993, -174.674)
  line L3517 (19.8574, -174.5626) -> (19.8387, -174.5276)
  arc A208 (1.2372, -67.0197) -> (1.92, -66.7368) centre (1.52, -66.7368) ccw
  line L3518 (20.0369, -174.4741) -> (20.012, -174.4275)
  line L3519 (1.92, -66.7368) -> (1.92, -64.6997)
  line L3520 (19.8993, -174.674) -> (19.8878, -174.636)
  line L3521 (-0.08, -54.8997) -> (-0.08, -65.0997)
  line L3522 (17.92, -57.4997) -> (17.92, -62.4997)
  line L3523 (19.8177, -174.4938) -> (19.7946, -174.4616)
  line L3524 (-0.0338, -65.4005) -> (-0.0174, -65.4367)
  line L3525 (19.8387, -174.5276) -> (19.8177, -174.4938)
  line L3526 (-0.2373, -65.4277) -> (-0.2187, -65.4771)
  line L3527 (-0.0478, -114.636) -> (-0.0593, -114.674)
  line L3528 (-0.0798, -74.2989) -> (-0.1133, -74.3397)
  line L3529 (3.2765, -75.2997) -> (1.92, -75.2997)
  line L3530 (-0.2786, -74.7804) -> (-0.28, -74.8985)
  line L3531 (-0.0478, -114.636) -> (-0.0593, -114.674)
  line L3532 (1.92, -122.4997) -> (1.92, -117.4997)
  line L3533 (-0.2732, -74.7258) -> (-0.2786, -74.7804)
  line L3534 (19.8738, -114.5988) -> (19.8574, -114.5626)
  line L3535 (19.9083, -114.7127) -> (19.8993, -114.674)
  line L3536 (5.2975, -80.1723) -> (5.348, -80.1569)
  line L3537 (16.0765, -117.4997) -> (17.92, -117.4997)
  line L3538 (5.1678, -79.9945) -> (5.207, -79.988)
  line L3539 (19.8993, -114.674) -> (19.8878, -114.636)
  line L3540 (20.0926, -114.6222) -> (20.0773, -114.5717)
  line L3541 (5.2457, -80.0203) -> (5.207, -80.0113)
  line L3542 (5.2457, -79.979) -> (5.2837, -79.9674)
  line L3543 (17.92, -117.4997) -> (17.92, -122.4997)
  line L3544 (5.246, -80.1843) -> (5.2975, -80.1723)
  line L3545 (5.207, -79.988) -> (5.2457, -79.979)
  line L3546 (5.348, -79.8424) -> (5.2975, -79.8271)
  line L3547 (19.9148, -114.7519) -> (19.9083, -114.7127)
  line L3548 (18.12, -115.4997) -> (16.4807, -115.4997)
  line L3549 (19.92, -114.8997) -> (19.9187, -114.7914)
  line L3550 (5.2975, -79.8271) -> (5.246, -79.8151)
  line L3551 (5.1939, -80.1929) -> (5.246, -80.1843)
  line L3552 (20.1186, -114.7804) -> (20.1132, -114.7258)
  line L3553 (5.207, -80.0113) -> (5.1678, -80.0049)
  line L3554 (16.1593, -117.2997) -> (18.12, -117.2997)
  line L3555 (5.3209, -80.0459) -> (5.2837, -80.0319)
  line L3556 (16.1593, -117.2997) -> (18.12, -117.2997)
  line L3557 (5.0918, -79.7997) -> (1.42, -79.7997)
  arc A209 (-0.28, -79.4997) -> (0.42, -80.1997) centre (0.42, -79.4997) ccw
  line L3558 (20.1132, -114.7258) -> (20.1046, -114.6736)
  line L3559 (19.92, -114.8997) -> (19.9187, -114.7914)
  line L3560 (5.4921, -80.0916) -> (5.537, -80.0637)
  line L3561 (5.2837, -79.9674) -> (5.3209, -79.9534)
  line L3562 (5.4888, -79.849) -> (5.5178, -79.8219)
  line L3563 (20.0773, -114.5717) -> (20.0587, -114.5222)
  line L3564 (17.92, -115.2997) -> (16.5635, -115.2997)
  line L3565 (19.8738, -114.5988) -> (19.8574, -114.5626)
  line L3566 (19.8574, -114.5626) -> (19.8387, -114.5276)
  line L3567 (18.12, -122.6997) -> (16.1593, -122.6997)
  line L3568 (5.5178, -80.1775) -> (5.4888, -80.1503)
  line L3569 (5.4888, -79.849) -> (5.5178, -79.8219)
  line L3570 (20.12, -114.8985) -> (20.1186, -114.7804)
  line L3571 (18.12, -115.4997) -> (16.4807, -115.4997)
  arc A210 (0.42, -79.9997) -> (-0.08, -80.4997) centre (0.42, -80.4997) ccw
  line L3572 (5.3209, -80.0459) -> (5.2837, -80.0319)
  line L3573 (5.5178, -80.1775) -> (5.4888, -80.1503)
  line L3574 (5.2837, -79.9674) -> (5.3209, -79.9534)
  line L3575 (19.8574, -114.5626) -> (19.8387, -114.5276)
  line L3576 (5.537, -79.9356) -> (5.4921, -79.9077)
  line L3577 (1.42, -79.9997) -> (0.42, -79.9997)
  arc A211 (18.6028, -112.9797) -> (17.92, -113.2625) centre (18.32, -113.2625) ccw
  arc A212 (-0.08, -79.4997) -> (0.42, -79.9997) centre (0.42, -79.4997) ccw
  line L3578 (19.9841, -114.3827) -> (19.9533, -114.3397)
  line L3579 (19.9198, -114.2989) -> (19.8859, -114.2627)
  line L3580 (19.8859, -114.2627) -> (18.6028, -112.9797)
  line L3581 (5.0886, -79.9997) -> (1.42, -79.9997)
  line L3582 (1.42, -79.9997) -> (5.0886, -79.9997)
  line L3583 (5.0886, -79.9997) -> (1.42, -79.9997)
  line L3584 (19.7694, -114.4308) -> (19.7422, -114.4019)
  line L3585 (0.42, -80.1997) -> (1.42, -80.1997)
  line L3586 (19.7694, -114.4308) -> (19.7422, -114.4019)
  line L3587 (1.42, -80.1997) -> (5.0918, -80.1997)
  line L3588 (19.8177, -114.4938) -> (19.7946, -114.4616)
  line L3589 (0.42, -79.9997) -> (1.42, -79.9997)
  line L3590 (19.9533, -114.3397) -> (19.9198, -114.2989)
  arc A213 (18.4614, -113.1211) -> (18.12, -113.2625) centre (18.32, -113.2625) ccw
  line L3591 (20.0369, -114.4741) -> (20.012, -114.4275)
  line L3592 (1.42, -79.7997) -> (0.42, -79.7997)
  arc A214 (18.4614, -113.1211) -> (18.12, -113.2625) centre (18.32, -113.2625) ccw
  line L3593 (20.012, -114.4275) -> (19.9841, -114.3827)
  line L3594 (0.42, -79.9997) -> (1.42, -79.9997)
  arc A215 (0.42, -79.9997) -> (-0.08, -80.4997) centre (0.42, -80.4997) ccw
  arc A216 (-0.08, -79.4997) -> (0.42, -79.9997) centre (0.42, -79.4997) ccw
  arc A217 (0.42, -79.7997) -> (-0.28, -80.4997) centre (0.42, -80.4997) ccw
  line L3595 (5.0886, -79.9997) -> (5.1283, -79.9984)
  line L3596 (1.42, -79.9997) -> (5.0886, -79.9997)
  line L3597 (19.7422, -114.4019) -> (18.4614, -113.1211)
  line L3598 (5.0886, -79.9997) -> (5.1283, -79.9984)
  line L3599 (1.42, -79.9997) -> (0.42, -79.9997)
  line L3600 (5.1413, -79.8013) -> (5.0918, -79.7997)
  line L3601 (5.0918, -80.1997) -> (5.1413, -80.198)
  line L3602 (5.1283, -80.001) -> (5.0886, -79.9997)
  line L3603 (19.7946, -114.4616) -> (19.7694, -114.4308)
  line L3604 (19.7422, -114.4019) -> (18.4614, -113.1211)
  line L3605 (19.8177, -114.4938) -> (19.7946, -114.4616)
  line L3606 (5.1283, -80.001) -> (5.0886, -79.9997)
  line L3607 (19.7946, -114.4616) -> (19.7694, -114.4308)
  line L3608 (13.6201, -109.9997) -> (13.82, -109.7998)
  line L3609 (9.713, -113.8997) -> (9.92, -113.6927)
  line L3610 (13.82, -112.839) -> (13.82, -110.1995)
  line L3611 (6.02, -72.839) -> (3.3593, -75.4997)
  line L3612 (13.82, -110.1995) -> (13.6201, -109.9997)
  line L3613 (9.92, -113.6927) -> (10.127, -113.8997)
  line L3614 (1.72, -75.4997) -> (1.72, -73.2625)
  line L3615 (13.82, -110.1995) -> (13.6201, -109.9997)
  circle A218 centre (9.92, -109.9997) radius 2.1
  line L3616 (9.713, -113.8997) -> (9.92, -113.6927)
  line L3617 (1.92, -75.2997) -> (1.92, -73.2625)
  line L3618 (6.02, -72.839) -> (3.3593, -75.4997)
  line L3619 (14.02, -112.7562) -> (14.02, -110.1167)
  line L3620 (10.0441, -114.0997) -> (12.6765, -114.0997)
  arc A219 (6.7986, -78.5411) -> (6.6572, -78.1997) centre (6.6572, -78.3997) ccw
  circle A220 centre (9.92, -109.9997) radius 2.1
  line L3621 (9.7959, -114.0997) -> (9.92, -113.9755)
  line L3622 (13.6201, -109.9997) -> (13.82, -109.7998)
  line L3623 (10.127, -113.8997) -> (12.7593, -113.8997)
  line L3624 (9.92, -113.9755) -> (10.0441, -114.0997)
  line L3625 (4.42, -76.5603) -> (7.0807, -73.8997)
  line L3626 (4.42, -76.5603) -> (7.0807, -73.8997)
  line L3627 (10.127, -113.8997) -> (12.7593, -113.8997)
  line L3628 (4.62, -77.9997) -> (4.62, -76.6432)
  line L3629 (3.3593, -75.4997) -> (1.72, -75.4997)
  arc A221 (6.7986, -78.5411) -> (6.6572, -78.1997) centre (6.6572, -78.3997) ccw
  line L3630 (5.82, -72.7562) -> (3.2765, -75.2997)
  line L3631 (13.903, -109.9997) -> (14.02, -109.8826)
  line L3632 (6.6572, -78.1997) -> (4.42, -78.1997)
  line L3633 (16.5635, -115.2997) -> (14.02, -112.7562)
  line L3634 (3.3593, -75.4997) -> (1.72, -75.4997)
  line L3635 (13.82, -112.839) -> (13.82, -110.1995)
  line L3636 (17.92, -113.2625) -> (17.92, -115.2997)
  arc A222 (1.72, -73.2625) -> (1.3786, -73.1211) centre (1.52, -73.2625) ccw
  line L3637 (18.12, -113.2625) -> (18.12, -115.4997)
  line L3638 (1.72, -75.4997) -> (1.72, -73.2625)
  line L3639 (12.6765, -114.0997) -> (16.0765, -117.4997)
  line L3640 (18.12, -113.2625) -> (18.12, -115.4997)
  line L3641 (12.7593, -113.8997) -> (16.1593, -117.2997)
  line L3642 (16.4807, -115.4997) -> (13.82, -112.839)